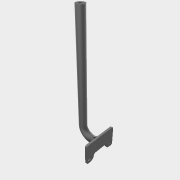
# Autodesk Inventor part: PWTR-0140
Saved by Autodesk Inventor 2021.1 (Build 251245000, 245)
## iProperties
Created: 2020-09-03
Part Number: PWTR-0140
Material: Steel
Document SubType Name: Modeling
Designer: alid
Density: 7.85 g/cm^3
Appearance: Smooth - Black
Description: Lifting Arm
Mass: 993.647 g
Surface Area: 325.007 cm^2
Volume: 126.579 cm^3
Author: alid
Revision Number: A
Autodesk Inventor part; units mm, degrees
ref_plane "YZ Plane" through (0, 0, 0) normal (1, 0, 0) x (0, 1, 0)
ref_plane "XZ Plane" through (0, 0, 0) normal (0, 1, 0) x (-1, 0, 0)
ref_plane "XY Plane" through (0, 0, 0) normal (0, 0, 1) x (1, 0, 0)
sketch "Sketch1" plane through (0, 0, 0) normal (0, 1, 0) x (-1, 0, 0)
  line L0 (42.5, -12.5) -> (-42.5, -12.5)
  line L1 (-42.5, -12.5) -> (-42.5, 12.5)
  line L2 (-42.5, 12.5) -> (42.5, 12.5)
  line L3 (42.5, 12.5) -> (42.5, -12.5)
  line L4 (-33.5, 0) -> (33.5, 0)
  line L5 (-42.5, -12.5) -> (-42.5, -30.5)
  line L6 (-42.5, -30.5) -> (-22.5, -30.5)
  line L7 (-22.5, -30.5) -> (-19.3261, -12.5)
  line L8 (-33.5, 0) -> (-33.5, -20)
  point P0 (0, 0)
  point P1 (42.5, 0)
  point P2 (0, 12.5)
  point P3 (0, 0)
  dimension "d0" = 85
  dimension "d1" = 25
  dimension "d10" = 67
  dimension "d31" = 18
  dimension "d32" = 20
  dimension "d33" = 100
  dimension "d36" = 20
  constraints: 18 end point, 3 midpoint, 2 horizontal, 2 parallel, 2 perpendicular, 2 vertical, 1 coincident, 1 horizontal alignment, 1 point on line, 1 vertical alignment
  measures "d0" distance of L1.end L2.end
  measures "d1" distance of L2.end L0.start
  measures "d10" distance of L4.start L4.end
  measures "d31" distance of L0.end L5.end
  measures "d32" distance of L5.end L6.end
  measures "d33" angle of L6 L7
  measures "d36" distance of L4.start L8.end
extrude "Extrusion1" add sketch "Sketch1" against normal blind 5 contours L0 L1 L2 L3
extrude "Extrusion3" add sketch "Sketch1" against normal up to surface (5 mm away) contours L7 L6 L5 L0
hole "Hole3" at (33.5, 0, -20) direction (0, -1, 0) diameter 8 end through all
mirror "Mirror1" about plane through (0, 0, 0) normal (1, 0, 0) of "Extrusion3", "Hole3"
sketch "Sketch2" plane through (0, 0, 0) normal (1, 0, 0) x (0, 1, 0)
  line L0 (0, 0) -> (25, 0)
  line L1 (50, 25) -> (50, 300)
  arc A0 (25, 0) -> (50, 25) centre (25, 25) ccw
  point P0 (50, 0)
  dimension "d4" = 300
  dimension "d5" = 50
  dimension "d6" = 25
  constraints: 4 end point, 2 point on circle, 2 point on line, 2 tangent, 1 centre point, 1 horizontal, 1 perpendicular
  measures "d4" distance of point (50, 0) L1.end
  measures "d5" distance of L0.start point (50, 0)
  measures "d6" radius of A0
sketch "Sketch3" plane through (0, 0, 0) normal (0, 1, 0) x (-1, 0, 0)
  circle A0 centre (0, 0) radius 10
  dimension "d7" = 20
  constraints: 1 centre point, 1 coincident
  measures "d7" diameter of A0
sweep "Sweep1" add profiles "Sketch3" path "Sketch2" path curves L0 A0 L1
sketch "Sketch6" plane through (0, 50, 300) normal (0, 0, 1) x (1, 0, 0)
  circle A0 centre (0, 0) radius 10 projected
  point P0 (0, -50)
  constraints: 1 coincident
hole "Hole4" at (0, 50, 300) direction (0, 0, -1) diameter 7.7978 depth 26.988 tip angle 118
move faces "Move1" translate (0, 0, 15) faces at (-14.1667, -1.6667, 12.5)
sketch "Sketch7" plane through (0, 0, 0) normal (0, 0, 1) x (1, 0, 0)
  line L0 (0, 0) -> (25, 0) construction
  line L1 (25, 0) -> (11.5003, 16.0883)
  dimension "d55" = 25
  dimension "d56" = 50
  constraints: 4 end point, 1 horizontal
  measures "d55" distance of L0.start L0.end
  measures "d56" angle of L0 L1
extrude "Rib1" add sketch "Sketch7" along normal mid plane 3 rib yes fills toward (18.2118, 8.012) open curves L1
pattern_circular "Circular Pattern1" count 3 over 180 about axis through (0, 0, 0) along (0, -1, 0) of "Rib1"
fillet "Fillet2" radius 5 6 edges at (42.5, -2.5, -30.5) (42.5, -2.5, 27.5) (19.3261, -2.5, -12.5) (-19.3261, -2.5, -12.5) (-42.5, -2.5, -30.5) (-42.5, -2.5, 27.5)
fillet "Fillet2" radius 12 2 edges at (22.5, -2.5, -30.5) (-22.5, -2.5, -30.5)
body "Solid1"
